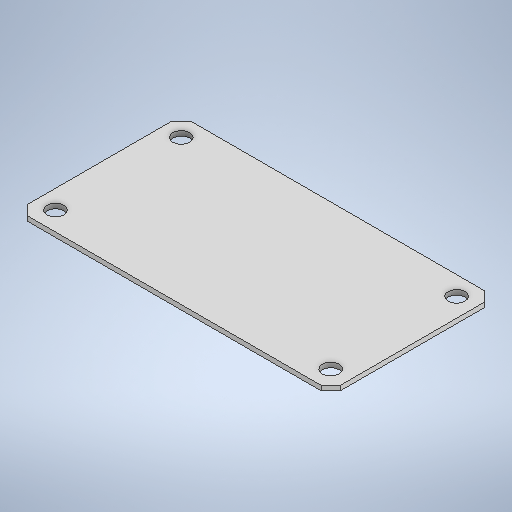
# Autodesk Inventor part: Extender
Saved by Autodesk Inventor 2025.2 (Build 292293000, 293)
## iProperties
Created: 2025-04-29
Part Number: Extender
Material: Generic
Document SubType Name: Sheet Metal
Designer: Caspe
Density: 1 g/cm^3
Sheet Metal Rule: Default_mm
Appearance: Default
Flat Pattern Width: 10.4 cm
Flat Pattern Length: 19.9 cm
Flat Pattern Area: 206.96 cm^2
Sheet Metal Width: 104,000 mm
Sheet Metal Length: 199,000 mm
Sheet Metal Area: 20696,000 mm^2
Author: Caspe
Autodesk Inventor part; units mm, degrees
ref_plane "YZ Plane" through (0, 0, 0) normal (1, 0, 0) x (0, 1, 0)
ref_plane "XZ Plane" through (0, 0, 0) normal (0, 1, 0) x (-1, 0, 0)
ref_plane "XY Plane" through (0, 0, 0) normal (0, 0, 1) x (1, 0, 0)
sketch "Sketch1" plane through (0, 0, 0) normal (0, 1, 0) x (-1, 0, 0)
  line L0 (0, 0) -> (-175, 0)
  line L1 (-175, 0) -> (-175, -80)
  line L2 (-175, -80) -> (0, -80)
  line L3 (0, -80) -> (0, 0)
  circle A0 centre (0, 0) radius 5.35
  circle A1 centre (0, -80) radius 5.35
  circle A2 centre (-175, -80) radius 5.35
  circle A3 centre (-175, 0) radius 5.35
  line L4 (12, 12) -> (-187, 12)
  line L5 (-187, 12) -> (-187, -92)
  line L6 (-187, -92) -> (12, -92)
  line L7 (12, -92) -> (12, 12)
  dimension "d0" = 175
  dimension "d1" = 80
  dimension "d2" = 10.7
  dimension "d3" = 10.7
  dimension "d4" = 10.7
  dimension "d5" = 10.7
  dimension "d6" = 12
  dimension "d7" = 12
  dimension "d8" = 12
  dimension "d9" = 12
  measures "d0" distance of L2.end L1.end
  measures "d1" distance of L1.end L0.end
  measures "d2" diameter of A0
  measures "d3" diameter of A1
  measures "d4" diameter of A2
  measures "d5" diameter of A3
  measures "d6" distance between parallel lines of L3 L7
  measures "d7" distance between parallel lines of L0 L4
  measures "d8" distance between parallel lines of L5 L1
  measures "d9" distance between parallel lines of L6 L2
extrude "Plate1" add sketch "Sketch1" along normal blind 3 contours L0 A0 L3 A1 L2 A2 L1 A3 | L7 L6 L5 L4
chamfer "Corner Chamfer1" distance 6 angle 45 4 edges at (-12, 1.5, 12) (187, 1.5, 12) (187, 1.5, -92) (-12, 1.5, -92)
equation "\"d3\" = d2"
equation "\"d4\" = d2"
equation "\"d5\" = d2"
equation "\"d7\" = d6"
equation "\"d8\" = d6"
equation "\"d9\" = d8"
equation "\"d10\" = Thickness"
equation "\"BendRadius\" = Thickness"
equation "\"BendReliefWidth\" = Thickness"
equation "\"BendReliefDepth\" = 0.5 * Thickness"
equation "\"CornerReliefSize\" = 4 * Thickness"
equation "\"MinimumRemnant\" = 2 * Thickness"
equation "\"TransitionRadius\" = BendRadius"
equation "\"JacobiRadiusSize\" = BendRadius"
equation "\"GapSize\" = Thickness"
equation "\"Thickness\" = 3"
body "Solid1"
